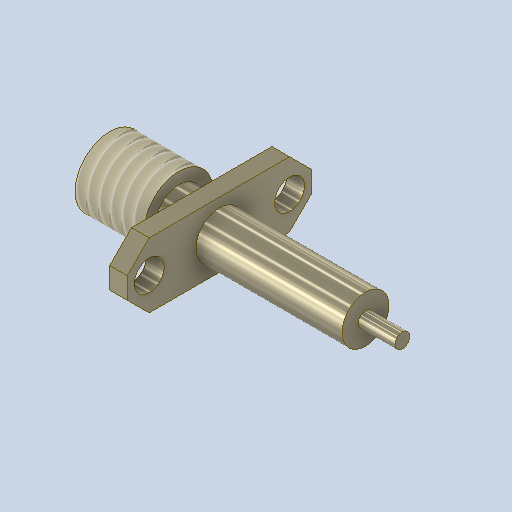
# Autodesk Inventor part: SMAPanel1
Saved by Autodesk Inventor 2026 (Build 300175050, 175E)
## iProperties
Created: 2018-08-15
Part Number: SMAPanel1
Material: Brass, Soft Yellow
Document SubType Name: Modeling
Designer: schanen
Density: 8.47 g/cm^3
Appearance: Nickel
Mass: 4.18807 g
Surface Area: 5.74005 cm^2
Volume: 0.4743 cm^3
Author: schanen
Autodesk Inventor part; units mm, degrees
ref_plane "YZ Plane" through (0, 0, 0) normal (1, 0, 0) x (0, 1, 0)
ref_plane "XZ Plane" through (0, 0, 0) normal (0, 1, 0) x (-1, 0, 0)
ref_plane "XY Plane" through (0, 0, 0) normal (0, 0, 1) x (1, 0, 0)
sketch "Sketch1" plane through (0, 0, 0) normal (1, 0, 0) x (0, 1, 0)
  line L0 (-2.825, 8) -> (2.825, 8)
  line L1 (2.825, 8) -> (2.825, -8)
  line L2 (2.825, -8) -> (-2.825, -8)
  line L3 (-2.825, -8) -> (-2.825, 8)
  line L4 (-2.825, 8) -> (2.825, -8) construction
  line L5 (2.825, 8) -> (-2.825, -8) construction
  point P0 (0, 0)
  dimension "d0" = 5.65
  dimension "d1" = 16
  constraints: 12 end point, 2 midpoint, 2 parallel, 1 horizontal, 1 perpendicular
  measures "d0" distance of L1.end L2.end
  measures "d1" distance of L0.end L1.end
extrude "Extrusion1" add sketch "Sketch1" along normal blind 1.53
sketch "Sketch2" plane through (1.53, 0, 0) normal (1, 0, 0) x (0, 0, -1)
  line L0 (8, 2.825) -> (-8, 2.825) projected
  line L1 (-6.1, -2.825) -> (6.1, -2.825)
  line L2 (6.1, -2.825) -> (6.1, 2.825) construction
  line L3 (6.1, 2.825) -> (-6.1, 2.825)
  line L4 (-6.1, 2.825) -> (-6.1, -2.825) construction
  line L5 (-6.1, -2.825) -> (6.1, 2.825) construction
  line L6 (6.1, -2.825) -> (-6.1, 2.825) construction
  point P0 (0, 0)
  point P1 (6.1, 0)
  point P2 (-6.1, 0)
  dimension "d4" = 12.2
  constraints: 12 end point, 4 midpoint, 2 parallel, 1 horizontal, 1 perpendicular, 1 point on line
  measures "d4" distance of L3.end L2.end
hole "Hole1" at (1.53, 0, -6.1) at (1.53, 0, 6.1) direction (-1, 0, 0) diameter 2.6 end through all
chamfer "Chamfer1" distance 1.9 angle 45 4 edges at (0.765, 2.825, 8) (0.765, 2.825, -8) (0.765, -2.825, 8) (0.765, -2.825, -8)
sketch "Sketch3" plane through (1.53, 0, 0) normal (1, 0, 0) x (0, 0, -1)
  circle A0 centre (0, 0) radius 2.03
  dimension "d15" = 4.06
  constraints: 1 centre point, 1 coincident
  measures "d15" diameter of A0
extrude "Extrusion2" add sketch "Sketch3" along normal blind 12.7
sketch "Sketch4" plane through (14.23, 0, 0) normal (1, 0, 0) x (0, 0, -1)
  circle A0 centre (0, 0) radius 0.6375
  dimension "d18" = 1.275
  constraints: 1 centre point, 1 coincident
  measures "d18" diameter of A0
extrude "Extrusion3" add sketch "Sketch4" along normal blind 3.2
sketch "Sketch5" plane through (0, 0, 0) normal (-1, 0, 0) x (0, 0, 1)
  circle A0 centre (0, 0) radius 2
  dimension "d21" = 4
  constraints: 1 centre point, 1 coincident
  measures "d21" diameter of A0
extrude "Extrusion4" add sketch "Sketch5" along normal blind 2
sketch "Sketch6" plane through (-2, 0, 0) normal (-1, 0, 0) x (0, 0, 1)
  circle A0 centre (0, 0) radius 3
  dimension "d24" = 6
  constraints: 1 centre point, 1 coincident
  measures "d24" diameter of A0
extrude "Extrusion5" add sketch "Sketch6" along normal blind 6
thread "Thread1" size "M6x1" class "6g" standard "ANSI Metric M Profile" full length
sketch "Sketch7" plane through (-8, 0, 0) normal (-1, 0, 0) x (0, 0, 1)
  circle A0 centre (0, 0) radius 0.6375 projected
  constraints: 1 coincident
hole "Hole2" at (-8, 0, 0) direction (1, 0, 0) diameter 0.7294 depth 3.5 tip angle 118 thread size "M1x0.25" class "6H" standard "ANSI Metric M Profile"
sketch "Sketch8" plane through (-8, 0, 0) normal (-1, 0, 0) x (0, 0, 1)
  circle A0 centre (0, 0) radius 0.3647 projected
  circle A1 centre (0, 0) radius 2.5
  dimension "d36" = 5
  constraints: 1 centre point, 1 coincident
  measures "d36" diameter of A1
extrude "Extrusion6" cut sketch "Sketch8" against normal blind 2
body "Solid1"
